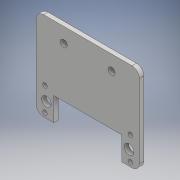
# Autodesk Inventor part: Support de 29mm Partie Basse
Saved by Autodesk Inventor 2017 (Build 210142000, 142)
## iProperties
Part Number: Support de 29mm Partie Basse
Material: Générique
Document SubType Name: Modeling
Designer: sasha
Density: 1 g/cm^3
Appearance: Par défaut
Author: sasha
Autodesk Inventor part; units mm, degrees
ref_plane "YZ Plane" through (0, 0, 0) normal (1, 0, 0) x (0, 1, 0)
ref_plane "XZ Plane" through (0, 0, 0) normal (0, 1, 0) x (-1, 0, 0)
ref_plane "XY Plane" through (0, 0, 0) normal (0, 0, 1) x (1, 0, 0)
sketch "Esquisse1" plane through (0, 0, 0) normal (0, 1, 0) x (-1, 0, 0)
  line L0 (0, 0) -> (70, 0)
  line L1 (70, 0) -> (70, -60)
  line L2 (70, -60) -> (0, -60)
  line L3 (0, -60) -> (0, 0)
  line L4 (58, 0) -> (65, 0)
  line L5 (70, -5) -> (70, -55)
  line L6 (65, -60) -> (5, -60)
  line L7 (0, -5) -> (0, -55)
  circle A0 centre (63, -50) radius 3.25
  circle A1 centre (51.22, -10) radius 2.3
  line L8 (35, -60) -> (35, 0) construction
  line L9 (12, -60) -> (58, -60)
  line L10 (58, -60) -> (58, -44)
  line L11 (58, -44) -> (12, -44)
  line L12 (12, -44) -> (12, -60)
  circle A2 centre (7, -50) radius 3.25
  circle A3 centre (18.78, -10) radius 2.3
  point P0 (18.78, -10)
  dimension "d0" = 60
  dimension "d1" = 70
  dimension "d2" = 10
  dimension "d3" = 7
  dimension "d4" = 18.78
  dimension "d5" = 18.78
  dimension "d6" = 10
  dimension "d7" = 10
  dimension "d8" = 6.5
  dimension "d9" = 4.6
  dimension "d10" = 35
  dimension "d11" = 12
  dimension "d12" = 12
  dimension "d13" = 16
  constraints: 26 end point, 4 centre point, 4 collinear, 4 parallel, 3 coincident, 2 horizontal, 2 midpoint, 2 perpendicular, 2 symmetric about line, 1 point on line, 2 other
  measures "d0" distance between parallel lines of L2 L0
  measures "d1" distance between parallel lines of L7 L1
  measures "d2" distance from line of L2 point (63, -50)
  measures "d3" horizontal distance of L5.end point (63, -50)
  measures "d4" distance from line of L1 point (51.22, -10)
  measures "d5" distance from line of L3 point (18.78, -10)
  measures "d6" distance from line of L0 point (51.22, -10)
  measures "d7" distance from line of L0 point (18.78, -10)
  measures "d8" diameter of A0
  measures "d9" diameter of A1
  measures "d10" distance between parallel lines of L7 L8
  measures "d11" distance between parallel lines of L1 L10
  measures "d12" distance between parallel lines of L7 L12
  measures "d13" distance between parallel lines of L9 L11
extrude "Extrusion1" add sketch "Esquisse1" along normal blind 3 contours L0 L1 L2 L10 L11 L12 L3
fillet "Congé1" radius 5 2 edges at (0, 1.5, 0) (-70, 1.5, 0)
fillet "Congé2" radius 5 2 edges at (0, 1.5, -60) (-70, 1.5, -60)
sketch "Esquisse2" plane through (0, 3, 0) normal (0, 1, 0) x (1, 0, 0)
  line L0 (0, 5) -> (0, 55) projected
  line L1 (0, 41) -> (-70, 41)
  line L2 (-70, 5) -> (-70, 55) projected
  line L3 (-5, 60) -> (-12, 60) projected
  line L4 (-12, 44) -> (-58, 44) projected
  line L5 (-35, 44) -> (-35, 0)
  line L6 (-65, 0) -> (-5, 0) projected
  line L7 (-58, 60) -> (-65, 60) projected
  point P0 (0, 0)
  point P1 (-6, 41)
  point P2 (-64, 41)
  point P3 (-64, 57)
  point P4 (-6, 57)
  dimension "d18" = 19
  dimension "d19" = 6
  dimension "d27" = 3
  dimension "d28" = 6
  constraints: 4 end point, 3 point on line, 2 midpoint, 2 symmetric about line, 1 horizontal
  measures "d18" distance between parallel lines of L3 L1
  measures "d19" distance from line of L0 point (-6, 41)
  measures "d27" distance from line of L7 point (-64, 57)
  measures "d28" distance from line of L2 point (-64, 57)
hole "Perçage1" at (-6, 3, -41) at (-64, 3, -41) at (-6, 3, -57) at (-64, 3, -57) direction (0, -1, 0) diameter 3 end through all
